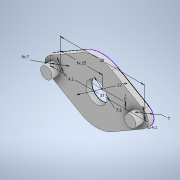
# Autodesk Inventor part: mount
Saved by Autodesk Inventor 2020 (Build 240168000, 168)
## iProperties
Created: 2021-11-22
Part Number: mount
Material: Generic
Document SubType Name: Modeling
Designer: bobox
Density: 1 g/cm^3
Appearance: Default
Author: bobox
Autodesk Inventor part; units mm, degrees
ref_plane "YZ Plane" through (0, 0, 0) normal (1, 0, 0) x (0, 1, 0)
ref_plane "XZ Plane" through (0, 0, 0) normal (0, 1, 0) x (-1, 0, 0)
ref_plane "XY Plane" through (0, 0, 0) normal (0, 0, 1) x (1, 0, 0)
sketch "Sketch1" plane through (0, 0, 0) normal (0, 0, 1) x (1, 0, 0)
  line L0 (0, 0) -> (30, 0) construction
  circle A0 centre (0, 0) radius 2.05
  circle A1 centre (30, 0) radius 2.05
  circle A2 centre (15, 0) radius 3.75
  line L1 (33.5, 0) -> (-3.5, 0) construction
  circle A3 centre (0, 0) radius 3.5 construction
  circle A4 centre (30, 0) radius 3.5 construction
  circle A5 centre (15, 0) radius 11 construction
  line L2 (-1.75, 3.0311) -> (9.5, 9.5263)
  line L3 (-1.75, -3.0311) -> (9.5, -9.5263)
  line L4 (20.5, -9.5263) -> (31.75, -3.0311)
  line L5 (31.75, 3.0311) -> (20.4846, 9.5352)
  arc A6 (-1.75, 3.0311) -> (-1.75, -3.0311) centre (0, 0) ccw
  arc A7 (20.4846, 9.5352) -> (9.5, 9.5263) centre (15, 0) ccw
  arc A8 (31.75, -3.0311) -> (31.75, 3.0311) centre (30, 0) ccw
  arc A9 (9.5, -9.5263) -> (20.5, -9.5263) centre (15, 0) ccw
  point P0 (31.75, -3.0311)
  dimension "d0" = 30
  dimension "d1" = 4.1
  dimension "d2" = 4.1
  dimension "d3" = 15
  dimension "d4" = 7.5
  dimension "d7" = 37
  dimension "d8" = 7
  dimension "d9" = 7
  dimension "d12" = 22
  dimension "d13" = 0
  constraints: 18 point on circle, 14 tangent, 12 end point, 10 centre point, 5 coincident, 2 horizontal, 1 concentric
  measures "d0" distance of L0.start L0.end
  measures "d1" diameter of A0
  measures "d2" diameter of A1
  measures "d3" distance of L0.start A2.centre
  measures "d4" diameter of A2
  measures "d7" distance of L1.start L1.end
  measures "d8" diameter of A4
  measures "d9" diameter of A3
  measures "d12" diameter of A5
  measures "d13" distance from line of L0 A2.centre
extrude "Extrusion1" add sketch "Sketch1" along normal blind 2
extrude "Extrusion2" add sketch "Sketch1" along normal blind 5 contours A0 | A1
equation "\"d2\" = d1"
equation "\"d3\" = 0.5 * d0"
equation "\"d9\" = d8"
body "Solid1"
